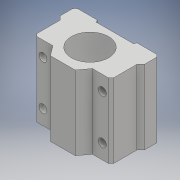
# Autodesk Inventor part: PilowBlockFechadoSCS8UU
Saved by Autodesk Inventor 2018 (Build 220112000, 112)
## iProperties
Created: 2018-09-20
Part Number: PilowBlockFechadoSCS8UU
Material: Genérico
Document SubType Name: Modeling
Designer: Georgines
Density: 1 g/cm^3
Appearance: Padrão
Author: Georgines
Autodesk Inventor part; units mm, degrees
ref_plane "YZ Plane" through (0, 0, 0) normal (1, 0, 0) x (0, 1, 0)
ref_plane "XZ Plane" through (0, 0, 0) normal (0, 1, 0) x (-1, 0, 0)
ref_plane "XY Plane" through (0, 0, 0) normal (0, 0, 1) x (1, 0, 0)
sketch "Esboço1" plane through (0, 0, 0) normal (0, 0, 1) x (1, 0, 0)
  line L0 (-17, 11) -> (17, 11) construction
  line L1 (17, 11) -> (17, -7) construction
  line L2 (17, -7) -> (-17, -7) construction
  line L3 (-17, -7) -> (-17, 11) construction
  line L4 (-14, 20.4248) -> (-14, -25.3484) construction
  line L5 (14, 20.4248) -> (14, -25.3484) construction
  line L6 (0, 20.9223) -> (0, -24.8509) construction
  line L7 (-26.3196, 0) -> (26.3196, 0) construction
  line L8 (-26.3196, 5) -> (26.3196, 5) construction
  line L9 (-15.5, 15.1736) -> (-15.5, -30.5996) construction
  line L10 (15.5, 20.4248) -> (15.5, -25.3484) construction
  line L11 (0, 0) -> (-21.4941, -25.6157) construction
  line L12 (0, 0) -> (11.7474, -14) construction
  line L13 (-8, 20.4248) -> (-8, -25.3484) construction
  line L14 (-5, 20.4248) -> (-5, -25.3484) construction
  line L15 (5, 20.9223) -> (5, -24.8509) construction
  line L16 (8, 20.9223) -> (8, -24.8509) construction
  line L17 (-26.3196, 3.5) -> (26.3196, 3.5) construction
  line L18 (-17, 11) -> (-17, 5)
  line L19 (-17, 5) -> (-15.5, 3.5)
  line L20 (-15.5, 3.5) -> (-15.5, -7)
  line L21 (17, 5) -> (17, 11)
  line L22 (26.3196, 10) -> (-26.3196, 10) construction
  line L23 (-17, 11) -> (-8, 11)
  line L24 (17, 11) -> (8, 11)
  line L25 (-8, 11) -> (-7.6714, 11) construction
  line L26 (-8, 11) -> (-7.5337, 10)
  line L27 (-8, 11) -> (-6.8966, 11) construction
  line L28 (-5, 11) -> (-3.8966, 11) construction
  line L29 (8, 11) -> (7.5337, 10)
  line L30 (15.5, -7) -> (15.5, 3.5)
  line L31 (17, 5) -> (15.5, 3.5)
  line L32 (-26.3196, -11) -> (26.3196, -11) construction
  line L33 (-7.5337, 10) -> (7.5337, 10)
  line L34 (-8, -7) -> (-5, -11)
  line L35 (8, -7) -> (5, -11)
  line L36 (-5, -11) -> (5, -11)
  line L37 (-8, -7) -> (-15.5, -7)
  line L38 (8, -7) -> (15.5, -7)
  circle A0 centre (0, 0) radius 7.5
  point P0 (0, 11)
  point P1 (0, 5)
  point P2 (0, -11)
  dimension "d0" = 34
  dimension "d1" = 18
  dimension "d2" = 14
  dimension "d3" = 14
  dimension "d4" = 11
  dimension "d5" = 6
  dimension "d6" = 1.5
  dimension "d7" = 1.5
  dimension "d8" = 40
  dimension "d9" = 40
  dimension "d10" = 5
  dimension "d11" = 5
  dimension "d12" = 8
  dimension "d13" = 8
  dimension "d14" = 1.5
  dimension "d15" = 1
  dimension "d18" = 115
  dimension "d20" = 115
  dimension "d21" = 22
  dimension "d22" = 15
  constraints: 78 end point, 31 point on line, 8 horizontal, 7 vertical, 6 parallel, 4 collinear, 4 midpoint, 3 coincident, 1 centre point, 1 equal length, 1 perpendicular
  measures "d0" distance of L0.start L0.end
  measures "d1" distance of L2.end L0.start
  measures "d2" distance between parallel lines of L4 L6
  measures "d3" distance between parallel lines of L5 L6
  measures "d4" distance between parallel lines of L7 L0
  measures "d5" distance between parallel lines of L8 L0
  measures "d6" distance between parallel lines of L1 L10
  measures "d7" distance between parallel lines of L3 L9
  measures "d8" angle of L11 L6
  measures "d9" angle of L6 L12
  measures "d10" distance between parallel lines of L14 L6
  measures "d11" distance between parallel lines of L15 L6
  measures "d12" distance between parallel lines of L13 L6
  measures "d13" distance between parallel lines of L16 L6
  measures "d14" distance between parallel lines of L17 L8
  measures "d15" distance between parallel lines of L22 L0
  measures "d18" angle of L29 L0
  measures "d20" angle of L26 L0
  measures "d21" distance between parallel lines of L32 L0
  measures "d22" diameter of A0
extrude "Extrusão1" add sketch "Esboço1" along normal blind 30
sketch "Esboço2" plane through (-17, 11, 0) normal (0, 1, 0) x (1, 0, 0)
  line L0 (0, 0) -> (0, -30) construction
  line L1 (0, -15) -> (34, -15) construction
  line L2 (34, 0) -> (34, -30) construction
  line L3 (17, 0) -> (17, -29.9375) construction
  circle A0 centre (5, -24) radius 1 construction
  circle A1 centre (5, -6) radius 1 construction
  circle A2 centre (29, -6) radius 1 construction
  circle A3 centre (29, -24) radius 1 construction
  dimension "d25" = 2
  dimension "d26" = 2
  dimension "d27" = 2
  dimension "d28" = 2
  dimension "d29" = 9
  dimension "d30" = 9
  dimension "d31" = 9
  dimension "d32" = 9
  dimension "d33" = 12
  dimension "d34" = 12
  dimension "d35" = 12
  dimension "d36" = 12
  constraints: 4 centre point, 4 end point, 2 midpoint, 1 vertical
  measures "d25" diameter of A0
  measures "d26" diameter of A1
  measures "d27" diameter of A2
  measures "d28" diameter of A3
  measures "d29" distance from line of L1 A1.centre
  measures "d30" distance from line of L1 A2.centre
  measures "d31" distance from line of L1 A3.centre
  measures "d32" distance from line of L1 A0.centre
  measures "d33" distance from line of L3 A1.centre
  measures "d34" distance from line of L3 A0.centre
  measures "d35" distance from line of L3 A3.centre
  measures "d36" distance from line of L3 A2.centre
hole "Furo1" at (-12, 11, 24) at (12, 11, 24) at (12, 11, 6) at (-12, 11, 6) direction (0, -1, 0) diameter 3.242 end through all thread size "M4x0.7" class "6H" standard "ANSI Metric M Profile"
chamfer "Chanfro1" distance 1 angle 45 4 edges at (-17, 11, 15) (17, 11, 15) (15.5, -7, 15) (-15.5, -7, 15)
equation "\"d3\" = d2"
equation "\"d7\" = d6"
equation "\"d9\" = d8"
equation "\"d11\" = d10"
equation "\"d13\" = d12"
equation "\"d26\" = d25"
equation "\"d27\" = d25"
equation "\"d28\" = d25"
equation "\"d30\" = d29"
equation "\"d31\" = d29"
equation "\"d32\" = d29"
equation "\"d34\" = d33"
equation "\"d35\" = d33"
equation "\"d36\" = d33"
